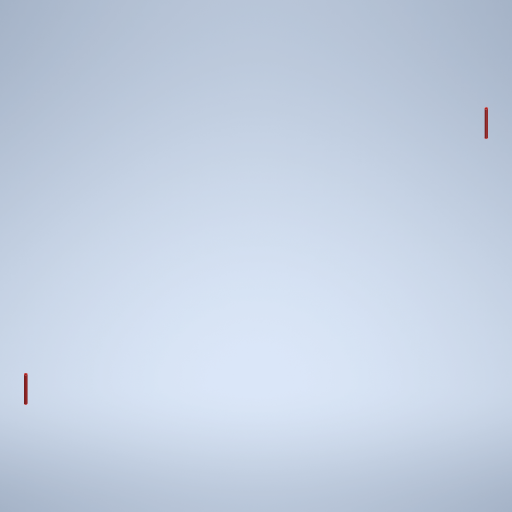
# Autodesk Inventor part: Minfix&Dowel Joint
Saved by Autodesk Inventor 2024 (Build 280153000, 153)
## iProperties
RuleStatus: InUse
Created: 2023-01-09
Part Number: Minfix&Dowel Joint
Material: Generic
Document SubType Name: Modeling
Designer: sauliusd
Density: 1 g/cm^3
Appearance: Default
AfterAnyUserParamChange0: ComponentsArrayParams
Author: sauliusd
Autodesk Inventor part; units mm, degrees
ref_plane "YZ Plane" through (0, 0, 0) normal (1, 0, 0) x (0, 1, 0)
ref_plane "XZ Plane" through (0, 0, 0) normal (0, 1, 0) x (-1, 0, 0)
ref_plane "XY Plane" through (0, 0, 0) normal (0, 0, 1) x (1, 0, 0)
sketch "Sketch1" plane through (0, 0, 0) normal (0, 0, 1) x (1, 0, 0)
  line L0 (-150, -10) -> (150, -10)
  line L1 (150, -10) -> (150, 10)
  line L2 (150, 10) -> (-150, 10)
  line L3 (-150, 10) -> (-150, -10)
  line L4 (-150, -10) -> (150, 10) construction
  line L5 (150, -10) -> (-150, 10) construction
  point P0 (0, 0)
  dimension "d0" = 300
  dimension "d1" = 20
  constraints: 12 end point, 2 midpoint, 2 parallel, 1 horizontal, 1 perpendicular
  measures "d0" distance of L2.end L1.end
  measures "d1" distance of L0.end L1.end
sketch "Lamello" plane through (0, 0, 0) normal (0, 0, 1) x (1, 0, 0)
  line L0 (50.583, 137.7858) -> (46.583, 137.7858)
  line L1 (46.583, 137.7858) -> (46.583, 113.1858)
  line L2 (46.583, 113.1858) -> (50.583, 113.1858)
  line L3 (50.583, 113.1858) -> (50.583, 137.7858)
  line L4 (50.583, 125.4858) -> (46.583, 125.4858)
  line L5 (48.583, 137.7858) -> (48.583, 113.1858)
  point P0 (48.583, 125.4858)
  dimension "LamelloGrooveThickness" = 4
  dimension "LamelloGrooveWidth" = 24.6
  measures "LamelloGrooveThickness" distance of L1.end L2.end
  measures "LamelloGrooveWidth" distance of L1.end L0.end
sketch "Sketch2" plane through (0, 0, 0) normal (0, 0, 1) x (1, 0, 0)
  circle A0 centre (90, 0) radius 0.5
  line L0 (150, 10) -> (-150, 10) projected
  line L1 (-150, -10) -> (150, -10) projected
  line L2 (0, -132.4) -> (0, 80.4) projected
  line L3 (150, -10) -> (150, 10) projected
  point P0 (0, 0)
  dimension "d4" = 1
  dimension "d50" = 10
  dimension "d70" = 60
  constraints: 1 centre point
  measures "d4" diameter of A0
  measures "d50" distance from line of L0 A0.centre
  measures "d70" distance from line of L3 A0.centre
extrude "Extrusion1" add sketch "Sketch2" along normal blind 10 contours A0
pattern_linear "Clamex Array" count 2 spacing 180 along (-1, 0, 0) of "Extrusion1"
sketch "Edge-Side Connection" plane through (0, 0, 0) normal (1, 0, 0) x (0, 1, 0)
  line L0 (-50, 0) -> (50, 0)
  line L1 (50, 0) -> (50, 18)
  line L2 (50, 18) -> (-50, 18)
  line L3 (-50, 18) -> (-50, 0)
  line L4 (-10, 0) -> (-10, -40)
  line L5 (-10, -40) -> (10, -40)
  line L6 (10, -40) -> (10, 0)
  line L7 (0, -12.3) -> (0, 15.7) construction
  line L8 (10, 0) -> (2, 0)
  line L9 (-2, -12.3) -> (-10, -12.3)
  point P0 (0, 0)
  point P1 (10, 0)
  point P2 (0, 0)
  dimension "d26" = 100
  dimension "d27" = 18
  dimension "d28" = 40
  dimension "OtherSideRefYCoordinate" = 10
  dimension "ReferenceCoord" = 10
  dimension "d49" = 90
  constraints: 20 end point, 4 parallel, 3 horizontal, 2 perpendicular, 2 point on line, 1 coincident, 1 midpoint, 1 vertical, 2 other
  measures "d26" distance of L2.end L1.end
  measures "d27" distance of L1.end L0.end
  measures "d28" distance between parallel lines of L0 L5
  measures "OtherSideRefYCoordinate" distance from line of point (-10, 0) L7
  measures "ReferenceCoord" distance from line of point (10, 0) L7
  measures "d49" angle of L6 L0
sketch "Edge-Edge Connection" plane through (0, 0, 0) normal (1, 0, 0) x (0, 1, 0)
  line L0 (-102, 18) -> (18, 18)
  line L1 (18, 18) -> (0, 0)
  line L2 (0, 0) -> (-102, 0)
  line L3 (-102, 0) -> (-102, 18)
  line L4 (18, 18) -> (18, -102)
  line L5 (0, 0) -> (0, -102)
  line L6 (0, -102) -> (18, -102)
  line L7 (2.6817, 2.6817) -> (0, 0)
  line L8 (-3.1873, 14.2075) -> (-3.1873, 18)
  point P0 (4.0959, 4.0959)
  dimension "d51" = 18
  dimension "d53" = 18
  dimension "EdgeEdgeReferenceCoord" = 5.7925
  dimension "d65" = 90
  dimension "d66" = 120
  dimension "d67" = 120
  dimension "EdgeEdgeOtherSideRefYCoordinate" = 19.6634
  constraints: 18 end point, 3 perpendicular, 2 parallel, 2 point on line, 1 coincident, 1 collinear, 1 equal length, 1 horizontal, 4 other
  measures "d51" distance between parallel lines of L2 L0
  measures "d53" distance between parallel lines of L4 L5
  measures "d65" angle of L2 L5
  measures "d66" distance of L0.start L0.end
  measures "d67" distance of L0.end L4.end
equation "\"d9\" = Step"
equation "\"d27\" = NestleBoardT"
equation "\"d0\" = ContactPatchWidth"
equation "\"d1\" = ContactPatchHeight"
equation "\"ContactPatchWidth\" = 300"
equation "\"ContactPatchHeight\" = 20"
equation "\"MinDistBetween\" = 96"
equation "\"Step\" = 180"
equation "\"NestleBoardT\" = 18"
equation "\"PillarBoardT\" = 18"
equation "\"AngleForYPositionCalc\" = 90deg"
equation "\"ConnectionAngle\" = 90deg"
equation "\"ShiftY\" = 0"
